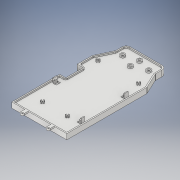
# Autodesk Inventor part: Display_Plate
Saved by Autodesk Inventor 2018 (Build 220112000, 112)
## iProperties
Created: 2019-05-28
Part Number: Display_Plate
Material: ABS Plastic
Document SubType Name: Modeling
Designer: Ash
Density: 1.06 g/cm^3
Appearance: Smooth - White
Author: Ash
Autodesk Inventor part; units mm, degrees
ref_plane "YZ Plane" through (0, 0, 0) normal (1, 0, 0) x (0, 1, 0)
ref_plane "XZ Plane" through (0, 0, 0) normal (0, 1, 0) x (-1, 0, 0)
ref_plane "XY Plane" through (0, 0, 0) normal (0, 0, 1) x (1, 0, 0)
sketch "Sketch1" plane through (0, 0, 0) normal (0, 1, 0) x (-1, 0, 0)
  line L0 (-80.01, -1.257939) -> (-80.01, -117.394059)
  line L1 (-80.01, -118.097939) -> (0, -118.097939) construction
  line L2 (0, -117.394059) -> (0, -96.380939)
  line L3 (-79.712527, -118.735872) -> (-69.512473, -140.609959)
  line L4 (-80.01, -118.097939) -> (-55.874615, -118.097939) construction
  line L5 (-0.297473, -118.735872) -> (-10.497527, -140.609959)
  line L6 (0, -118.097939) -> (24.135385, -118.097939) construction
  line L7 (-10.795, -141.247892) -> (-69.215, -141.247892) construction
  line L8 (-69.215, -141.951772) -> (-69.215, -150.645892)
  line L9 (-62.865, -156.995892) -> (-17.145, -156.995892)
  line L10 (-10.795, -150.645892) -> (-10.795, -141.951772)
  arc A0 (-0.297473, -118.735872) -> (0, -117.394059) centre (-3.175, -117.394059) ccw
  arc A1 (-80.01, -117.394059) -> (-79.712527, -118.735872) centre (-76.835, -117.394059) ccw
  arc A2 (-69.215, -150.645892) -> (-62.865, -156.995892) centre (-62.865, -150.645892) ccw
  arc A3 (-17.145, -156.995892) -> (-10.795, -150.645892) centre (-17.145, -150.645892) ccw
  arc A4 (-10.497527, -140.609959) -> (-10.795, -141.951772) centre (-7.62, -141.951772) ccw
  arc A5 (-69.215, -141.951772) -> (-69.512473, -140.609959) centre (-72.39, -141.951772) ccw
  line L11 (0, -96.380939) -> (-8.763, -96.380939)
  line L12 (-8.763, -96.380939) -> (-8.763, -70.980939)
  line L13 (-8.763, -70.980939) -> (0, -70.980939)
  line L14 (-80.01, -1.257939) -> (0, -1.257939)
  line L15 (0, -70.980939) -> (0, -1.257939)
  point P0 (0, 0)
  point P1 (-69.215, -156.995892)
  dimension "d0" = 80.01
  dimension "d1" = 116.84
  dimension "d3" = 65
  dimension "d4" = 115
  dimension "d5" = 58.42
  dimension "d6" = 15.748
  dimension "d7" = 3.175
  dimension "d8" = 6.35
  dimension "d9" = 3.175
  dimension "d45" = 8.763
  dimension "d46" = 25.4
  dimension "d47" = 21.717
  constraints: 32 end point, 12 point on circle, 12 point on line, 12 tangent, 6 centre point, 5 horizontal, 4 parallel, 4 perpendicular, 3 equal radius, 2 equal length, 1 horizontal alignment, 1 vertical
  measures "d0" distance of L1.end L1.start
  measures "d1" distance of L0.start L1.start
  measures "d3" angle of L3 L4
  measures "d4" angle of L5 L6
  measures "d5" distance of point (-69.215, -141.248) L7.start
  measures "d6" distance of point (-69.215, -156.996) L7.end
  measures "d7" radius of A0
  measures "d8" radius of A2
  measures "d9" radius of A4
  measures "d45" distance of L2.end L11.end
  measures "d46" distance of L11.end L12.end
  measures "d47" distance from line of L1.end L11
extrude "Extrusion1" add sketch "Sketch1" along normal blind 3.81
shell "Shell1" thickness 1.778 removed faces 1 at (56.261, 3.81, -63.210979)
sketch "Sketch2" plane through (1.778, 1.778, -1.778) normal (0, 1, 0) x (1, 0, 0)
  arc A0 (65.659, 140.173772) -> (66.123058, 138.080544) centre (70.612, 140.173772) ccw
  line L0 (65.776406, 139.101747) -> (60.579, 139.101747)
  line L1 (65.659, 148.867892) -> (65.659, 140.173772)
  line L2 (65.659, 140.625747) -> (60.579, 140.625747)
  line L3 (76.454, 115.616059) -> (76.454, 1.257939)
  arc A1 (76.454, 115.616059) -> (76.323112, 116.206456) centre (75.057, 115.616059) ccw
  line L4 (66.123058, 138.080544) -> (76.323112, 116.206456)
  arc A2 (65.659, 140.173772) -> (66.123058, 138.080544) centre (70.612, 140.173772) ccw
  line L5 (65.659, 148.867892) -> (65.659, 140.173772)
  arc A3 (65.659, 148.867892) -> (61.087, 153.439892) centre (61.087, 148.867892) ccw construction
  line L6 (15.367, 153.439892) -> (61.087, 153.439892) construction
  arc A4 (15.367, 153.439892) -> (10.795, 148.867892) centre (15.367, 148.867892) ccw construction
  line L7 (10.795, 140.173772) -> (10.795, 148.867892)
  arc A5 (10.330942, 138.080544) -> (10.795, 140.173772) centre (5.842, 140.173772) ccw
  line L8 (0.130888, 116.206456) -> (10.330942, 138.080544) construction
  arc A6 (0.130888, 116.206456) -> (0, 115.616059) centre (1.397, 115.616059) ccw
  line L9 (0, 96.380939) -> (0, 115.616059)
  circle A7 centre (57.235739, 139.863747) radius 1.905
  circle A8 centre (57.235739, 139.863747) radius 3.429
  line L10 (65.776406, 139.863747) -> (47.229764, 139.863747) construction
  line L11 (15.367, 153.439892) -> (61.087, 153.439892) construction
  line L12 (38.227, 153.439892) -> (38.227, -24.551353) construction
  line L13 (57.235739, 139.863747) -> (57.235739, 153.439892) construction
  line L14 (56.473739, 143.207008) -> (56.473739, 153.439892)
  line L15 (57.997739, 143.211092) -> (57.997739, 153.439892)
  line L16 (57.235739, 139.863747) -> (38.227, 145.482717) construction
  line L17 (57.235739, 139.863747) -> (38.227, 132.020717) construction
  circle A9 centre (38.227, 132.020717) radius 1.905
  circle A10 centre (38.227, 145.482717) radius 1.905
  circle A11 centre (38.227, 132.020717) radius 3.429
  circle A12 centre (38.227, 145.482717) radius 3.429
  line L18 (41.649128, 145.265732) -> (54.245625, 141.542217)
  line L19 (59.516104, 139.968345) -> (54.495452, 137.802468) construction
  line L20 (41.217114, 143.804247) -> (53.813611, 140.080731)
  line L21 (54.950087, 139.741356) -> (53.872726, 139.19428) construction
  line L22 (53.813611, 140.080731) -> (54.950087, 139.741356) construction
  line L23 (53.872726, 139.19428) -> (41.064475, 133.946016)
  line L24 (54.245625, 141.542217) -> (59.516104, 139.968345) construction
  line L25 (54.495452, 137.802468) -> (41.618556, 132.526076)
  line L26 (10.677594, 139.101747) -> (15.875, 139.101747)
  line L27 (10.795, 140.625747) -> (15.875, 140.625747)
  circle A13 centre (19.218261, 139.863747) radius 1.905
  circle A14 centre (19.218261, 139.863747) radius 3.429
  line L28 (19.980261, 143.207008) -> (19.980261, 153.439892)
  line L29 (18.456261, 143.211092) -> (18.456261, 153.439892)
  line L30 (34.804872, 145.265732) -> (22.208375, 141.542217)
  line L31 (35.236886, 143.804247) -> (22.640389, 140.080731)
  line L32 (22.581274, 139.19428) -> (35.389525, 133.946016)
  line L33 (21.958548, 137.802468) -> (34.835444, 132.526076)
  line L34 (34.835444, 132.526076) -> (21.958548, 137.802468)
  line L35 (22.581274, 139.19428) -> (35.389525, 133.946016)
  circle A15 centre (38.227, 132.020717) radius 3.429
  circle A16 centre (38.227, 145.482717) radius 3.429
  circle A17 centre (19.218261, 139.863747) radius 3.429
  line L36 (15.367, 153.439892) -> (61.087, 153.439892)
  line L37 (8.763, 96.380939) -> (0, 96.380939)
  line L38 (8.763, 67.424939) -> (8.763, 96.380939)
  line L39 (0, 67.424939) -> (8.763, 67.424939)
  line L40 (0, 1.257939) -> (0, 67.424939)
  line L41 (76.454, 1.257939) -> (0, 1.257939)
  point P0 (-1.778, -1.778)
  dimension "d13" = 1.524
  dimension "d14" = 5.08
  dimension "d15" = 3.81
  dimension "d16" = 1.524
  dimension "d17" = 0.762
  dimension "d20" = 1.524
  dimension "d21" = 0.762
  dimension "d22" = 13.462
  dimension "d23" = 3.81
  dimension "d24" = 3.81
  dimension "d25" = 1.524
  dimension "d26" = 1.524
  dimension "d27" = 0.762
  dimension "d28" = 0.762
  dimension "d30" = 1.524
  constraints: 54 end point, 17 symmetric about line, 7 centre point, 7 point on line, 6 point on circle, 5 coincident, 4 parallel, 2 horizontal, 2 vertical, 1 concentric, 1 midpoint, 1 perpendicular, 28 other
  measures "d13" distance between parallel lines of L0 L2
  measures "d14" distance of L2.start L2.end
  measures "d15" diameter of A7
  measures "d17" distance between parallel lines of L0 L10
  measures "d20" distance between parallel lines of L15 L14
  measures "d21" distance between parallel lines of L13 L14
  measures "d22" distance of L16.end L17.end
  measures "d23" diameter of A9
  measures "d24" diameter of A10
  measures "d25" radial gap between concentric circles of A9 A11
  measures "d26" radial gap between concentric circles of A10 A12
  measures "d27" distance between parallel lines of L16 L18
  measures "d28" distance between parallel lines of L16 L20
  measures "d30" distance between parallel lines of L25 L23
sketch "Sketch3" plane through (1.778, 1.778, -1.778) normal (0, 1, 0) x (1, 0, 0)
  circle A0 centre (19.218261, 139.748807) radius 1.905
  circle A1 centre (19.218261, 139.748807) radius 3.429
  circle A2 centre (38.227, 145.482717) radius 1.905
  circle A3 centre (38.227, 145.482717) radius 3.429
  circle A4 centre (38.227, 132.020717) radius 1.905
  circle A5 centre (38.227, 132.020717) radius 3.429
  circle A6 centre (57.235739, 139.748807) radius 1.905
  circle A7 centre (57.235739, 139.748807) radius 3.429
  arc A8 (60.579, 140.510807) -> (60.579, 140.510807) centre (57.235739, 139.748807) ccw
  line L0 (58.00154, 143.0912) -> (58.00154, 153.324952)
  line L1 (15.367, 153.439892) -> (61.087, 153.439892)
  line L2 (56.471752, 153.324952) -> (56.471752, 143.091615)
  line L3 (65.659, 148.867892) -> (65.659, 140.173772)
  arc A9 (65.659, 148.867892) -> (61.087, 153.439892) centre (61.087, 148.867892) ccw
  line L4 (15.367, 153.439892) -> (61.087, 153.439892)
  arc A10 (15.367, 153.439892) -> (10.795, 148.867892) centre (15.367, 148.867892) ccw
  line L5 (10.795, 140.173772) -> (10.795, 148.867892)
  arc A11 (10.330942, 138.080544) -> (10.795, 140.173772) centre (5.842, 140.173772) ccw
  line L6 (0.130888, 116.206456) -> (10.330942, 138.080544)
  arc A12 (0.130888, 116.206456) -> (0, 115.616059) centre (1.397, 115.616059) ccw
  line L7 (0, 96.380939) -> (0, 115.616059)
  line L8 (76.454, 115.616059) -> (76.454, 1.257939)
  arc A13 (76.454, 115.616059) -> (76.323112, 116.206456) centre (75.057, 115.616059) ccw
  line L9 (66.123058, 138.080544) -> (76.323112, 116.206456)
  arc A14 (65.659, 140.173772) -> (66.123058, 138.080544) centre (70.612, 140.173772) ccw
  line L10 (18.476733, 153.439892) -> (18.476733, 143.211608)
  circle A15 centre (19.218261, 139.748807) radius 3.429
  line L11 (19.95979, 143.096669) -> (19.95979, 153.439892)
  line L12 (22.199011, 141.443851) -> (34.80613, 145.246738)
  arc A16 (41.656, 145.482717) -> (41.656, 145.482717) centre (38.227, 145.482717) ccw
  line L13 (35.24625, 143.787673) -> (22.639132, 139.984786)
  line L14 (22.022965, 137.776073) -> (34.835444, 132.526076)
  arc A17 (41.656, 132.020717) -> (41.656, 132.020717) centre (38.227, 132.020717) ccw
  line L15 (22.600805, 139.186277) -> (35.389525, 133.946016)
  line L16 (15.875, 140.510807) -> (10.795, 140.510807)
  line L17 (10.795, 140.173772) -> (10.795, 148.867892)
  line L18 (15.875, 138.986807) -> (10.677594, 139.101747)
  line L19 (8.763, 96.380939) -> (0, 96.380939)
  line L20 (8.763, 67.424939) -> (8.763, 96.380939)
  line L21 (0, 67.424939) -> (8.763, 67.424939)
  line L22 (0, 1.257939) -> (0, 67.424939)
  line L23 (76.454, 1.257939) -> (0, 1.257939)
  point P0 (-1.778, -1.778)
  constraints: 20 end point, 7 point on circle, 3 point on line, 2 parallel, 2 vertical, 1 horizontal, 1 perpendicular, 9 other
sketch "Sketch5" plane through (1.778, 1.778, -1.778) normal (0, 1, 0) x (1, 0, 0)
  line L0 (0, 96.380939) -> (0, 115.616059)
  line L1 (0, 115.616059) -> (10.16, 115.616059) construction
  arc A0 (76.454, 115.616059) -> (76.323112, 116.206456) centre (75.057, 115.616059) ccw
  line L2 (76.323112, 116.206456) -> (66.163112, 116.206456) construction
  line L3 (-1.778, 69.202939) -> (-1.778, -1.778)
  line L4 (-1.778, 23.137892) -> (19.304, 23.137892) construction
  line L5 (-1.778, 23.137892) -> (19.304, 23.137892) construction
  line L6 (76.454, 23.137892) -> (55.372, 23.137892) construction
  line L7 (61.087, 155.217892) -> (15.367, 155.217892)
  line L8 (9.496281, 155.217892) -> (45.056281, 155.217892) construction
  line L9 (10.795, 140.510807) -> (22.647261, 140.510807) construction
  line L10 (10.16, 116.378059) -> (5.08, 116.378059)
  line L11 (5.08, 116.378059) -> (5.08, 114.854059)
  line L12 (5.08, 114.854059) -> (10.16, 114.854059)
  line L13 (10.16, 114.854059) -> (10.16, 116.378059)
  line L14 (6.858, 113.076059) -> (8.382, 113.076059)
  line L15 (8.382, 113.076059) -> (8.382, 118.156059)
  line L16 (8.382, 118.156059) -> (6.858, 118.156059)
  line L17 (6.858, 118.156059) -> (6.858, 113.076059)
  line L18 (6.858, 113.076059) -> (8.382, 118.156059) construction
  line L19 (8.382, 113.076059) -> (6.858, 118.156059) construction
  line L20 (7.62, 116.378059) -> (7.62, 114.854059) construction
  circle A1 centre (7.62, 115.616059) radius 0.889
  line L21 (68.703112, 115.444456) -> (63.623112, 115.444456)
  line L22 (63.623112, 115.444456) -> (63.623112, 116.968456)
  line L23 (63.623112, 116.968456) -> (68.703112, 116.968456)
  line L24 (68.703112, 116.968456) -> (68.703112, 115.444456)
  line L25 (65.401112, 113.666456) -> (66.925112, 113.666456)
  line L26 (66.925112, 113.666456) -> (66.925112, 118.746456)
  line L27 (66.925112, 118.746456) -> (65.401112, 118.746456)
  line L28 (65.401112, 118.746456) -> (65.401112, 113.666456)
  line L29 (65.401112, 113.666456) -> (66.925112, 118.746456) construction
  line L30 (66.925112, 113.666456) -> (65.401112, 118.746456) construction
  line L31 (66.163112, 115.444456) -> (66.163112, 116.968456) construction
  circle A2 centre (66.163112, 116.206456) radius 0.889
  line L32 (54.61, 20.597892) -> (56.134, 20.597892)
  line L33 (55.372, 22.375892) -> (55.372, 23.899892) construction
  line L34 (52.832, 23.899892) -> (57.912, 23.899892)
  circle A3 centre (55.372, 23.137892) radius 0.889
  line L35 (57.912, 23.899892) -> (57.912, 22.375892)
  line L36 (57.912, 22.375892) -> (52.832, 22.375892)
  line L37 (56.134, 20.597892) -> (56.134, 25.677892)
  line L38 (54.61, 20.597892) -> (56.134, 25.677892) construction
  line L39 (56.134, 20.597892) -> (54.61, 25.677892) construction
  line L40 (54.61, 25.677892) -> (54.61, 20.597892)
  line L41 (56.134, 25.677892) -> (54.61, 25.677892)
  line L42 (52.832, 22.375892) -> (52.832, 23.899892)
  line L43 (18.542, 20.597892) -> (20.066, 20.597892)
  line L44 (19.304, 22.375892) -> (19.304, 23.899892) construction
  line L45 (16.764, 23.899892) -> (21.844, 23.899892)
  circle A4 centre (19.304, 23.137892) radius 0.889
  line L46 (21.844, 23.899892) -> (21.844, 22.375892)
  line L47 (21.844, 22.375892) -> (16.764, 22.375892)
  line L48 (20.066, 20.597892) -> (20.066, 25.677892)
  line L49 (18.542, 20.597892) -> (20.066, 25.677892) construction
  line L50 (20.066, 20.597892) -> (18.542, 25.677892) construction
  line L51 (18.542, 25.677892) -> (18.542, 20.597892)
  line L52 (20.066, 25.677892) -> (18.542, 25.677892)
  line L53 (16.764, 22.375892) -> (16.764, 23.899892)
  line L54 (76.454, 115.616059) -> (76.454, 1.257939)
  line L55 (76.454, 0) -> (0, 0)
  point P0 (22.647261, 139.748807)
  point P1 (68.703112, 117.203559)
  point P2 (57.912, 118.791059)
  point P3 (55.372, 23.137892)
  point P4 (21.844, 120.378559)
  point P5 (19.304, 23.137892)
  point P6 (7.62, 115.616059)
  dimension "d48" = 10.16
  dimension "d49" = 10.16
  dimension "d50" = 21.082
  dimension "d52" = 21.082
  dimension "d56" = 0.762
  dimension "d57" = 0.762
  dimension "d58" = 5.08
  dimension "d59" = 1.524
  dimension "d60" = 5.08
  dimension "d61" = 1.778
  dimension "d66" = 5.08
  dimension "d67" = 1.524
  dimension "d68" = 5.08
  dimension "d69" = 1.778
  dimension "d70" = 1.524
  dimension "d71" = 5.08
  dimension "d72" = 1.524
  dimension "d73" = 5.08
  dimension "d74" = 1.778
  dimension "d75" = 1.524
  dimension "d76" = 5.08
  dimension "d77" = 1.524
  dimension "d78" = 5.08
  dimension "d79" = 1.778
  dimension "d80" = 1.524
  dimension "d160" = 132.08
  constraints: 100 end point, 27 midpoint, 16 parallel, 12 horizontal, 9 perpendicular, 9 point on line, 4 centre point, 4 coincident, 1 collinear
  measures "d48" distance of L0.end L1.end
  measures "d49" distance of L2.start L2.end
  measures "d50" distance of L4.end L4.start
  measures "d52" distance of L6.end L6.start
  measures "d56" distance between parallel lines of L1 L10
  measures "d57" distance between parallel lines of L1 L12
  measures "d58" distance between parallel lines of L13 L11
  measures "d59" distance of L16.end L15.end
  measures "d60" distance of L15.end L14.end
  measures "d61" diameter of A1
  measures "d66" distance between parallel lines of L24 L22
  measures "d67" distance of L30.end L26.end
  measures "d68" distance of L26.end L25.end
  measures "d69" diameter of A2
  measures "d70" distance between parallel lines of L21 L23
  measures "d71" distance between parallel lines of L35 L42
  measures "d72" distance of L41.end L37.end
  measures "d73" distance of L37.end L32.end
  measures "d74" diameter of A3
  measures "d75" distance between parallel lines of L36 L34
  measures "d76" distance between parallel lines of L46 L53
  measures "d77" distance of L52.end L48.end
  measures "d78" distance of L48.end L43.end
  measures "d79" diameter of A4
  measures "d80" distance between parallel lines of L47 L45
  measures "d160" distance between parallel lines of L7 L6
extrude "Extrusion7" add sketch "Sketch5" along normal blind 3.048 contours A1 L15 L12 L17 L10 | L10 A1 | A1 L15 | A1 L12 | L17 A1 | A2 L21 | L21 A2 L28 L23 L26 | L26 A2 | L23 A2 | A2 L28 | L36 A3 | A3 L40 L34 L37 L36 | A3 L40 | L37 A3 | A3 L34 | L47 A4 | A4 L51 L45 L48 L47 | A4 L51 | L48 A4 | A4 L45
extrude "Extrusion8" add sketch "Sketch5" along normal up to surface (2.032 mm away)
sketch "Sketch6" plane through (1.778, 1.778, -1.778) normal (0, 1, 0) x (1, 0, 0)
  line L0 (3.302, 61.074939) -> (7.366, 61.074939)
  line L1 (7.366, 61.074939) -> (7.366, 54.978939)
  line L2 (7.366, 54.978939) -> (3.302, 54.978939)
  line L3 (3.302, 54.978939) -> (3.302, 61.074939)
  line L4 (0, 67.424939) -> (8.763, 67.424939)
  line L5 (6.985, 69.202939) -> (-1.778, 69.202939)
  line L6 (-1.778, 69.202939) -> (-1.778, -1.778)
  line L7 (69.088, 29.718) -> (73.152, 29.718)
  line L8 (73.152, 29.718) -> (73.152, 23.622)
  line L9 (73.152, 23.622) -> (69.088, 23.622)
  line L10 (69.088, 23.622) -> (69.088, 29.718)
  line L11 (78.232, -0.520061) -> (78.232, 115.616059)
  line L12 (-1.778, -1.778) -> (78.232, -1.778)
  line L13 (69.088, 93.218) -> (73.152, 93.218)
  line L14 (73.152, 93.218) -> (73.152, 87.122)
  line L15 (73.152, 87.122) -> (69.088, 87.122)
  line L16 (69.088, 87.122) -> (69.088, 93.218)
  line L17 (76.454, 115.616059) -> (76.454, 1.257939)
  point P0 (0, 67.31)
  point P1 (76.454, 0)
  dimension "d82" = 4.064
  dimension "d83" = 6.096
  dimension "d85" = 8.128
  dimension "d86" = 5.08
  dimension "d87" = 4.064
  dimension "d88" = 6.096
  dimension "d89" = 5.08
  dimension "d90" = 25.4
  dimension "d91" = 4.064
  dimension "d92" = 6.096
  dimension "d93" = 88.9
  dimension "d95" = 5.08
  constraints: 24 end point, 6 parallel, 3 horizontal, 3 perpendicular, 1 other
  measures "d82" distance of L1.end L2.end
  measures "d83" distance of L0.end L1.end
  measures "d85" distance between parallel lines of L5 L0
  measures "d86" distance between parallel lines of L6 L3
  measures "d87" distance of L8.end L9.end
  measures "d88" distance of L7.end L8.end
  measures "d89" distance between parallel lines of L11 L8
  measures "d90" distance between parallel lines of L12 L9
  measures "d91" distance of L14.end L15.end
  measures "d92" distance of L13.end L14.end
  measures "d93" distance between parallel lines of L12 L15
  measures "d95" distance between parallel lines of L11 L14
extrude "Extrusion9" cut sketch "Sketch6" against normal through all
sketch "Sketch7" plane through (1.778, 1.778, -1.778) normal (0, 1, 0) x (1, 0, 0)
  line L0 (3.302, 54.978939) -> (3.302, 61.074939)
  line L1 (3.302, 60.439939) -> (2.032, 60.439939)
  line L2 (2.032, 60.439939) -> (2.032, 55.486939)
  line L3 (2.032, 55.486939) -> (3.302, 55.486939)
  line L4 (3.302, 55.486939) -> (3.302, 60.439939)
  line L5 (3.302, 61.074939) -> (7.366, 61.074939)
  line L6 (74.422, 92.583) -> (73.152, 92.583)
  line L7 (73.152, 92.583) -> (73.152, 87.63)
  line L8 (73.152, 87.63) -> (74.422, 87.63)
  line L9 (74.422, 87.63) -> (74.422, 92.583)
  line L10 (73.152, 93.218) -> (73.152, 87.122)
  line L11 (69.088, 93.218) -> (73.152, 93.218)
  line L12 (74.422, 29.21) -> (73.152, 29.21)
  line L13 (73.152, 29.21) -> (73.152, 24.257)
  line L14 (73.152, 24.257) -> (74.422, 24.257)
  line L15 (74.422, 24.257) -> (74.422, 29.21)
  line L16 (73.152, 29.718) -> (73.152, 23.622)
  line L17 (69.088, 29.718) -> (73.152, 29.718)
  line L18 (73.152, 23.622) -> (69.088, 23.622)
  point P0 (-1.778, -1.778)
  dimension "d98" = 1.27
  dimension "d99" = 4.953
  dimension "d100" = 0.635
  dimension "d103" = 1.27
  dimension "d104" = 4.953
  dimension "d105" = 0.635
  dimension "d106" = 1.27
  dimension "d107" = 4.953
  dimension "d109" = 0.635
  constraints: 24 end point, 6 parallel, 3 horizontal, 3 perpendicular, 2 collinear, 1 point on line
  measures "d98" distance of L3.end L2.end
  measures "d99" distance of L2.end L1.end
  measures "d100" distance between parallel lines of L5 L1
  measures "d103" distance of L8.end L7.end
  measures "d104" distance of L7.end L6.end
  measures "d105" distance between parallel lines of L11 L6
  measures "d106" distance of L14.end L13.end
  measures "d107" distance of L13.end L12.end
  measures "d109" distance between parallel lines of L18 L14
extrude "Extrusion10" add sketch "Sketch7" along normal blind 6.604
sketch "Sketch8" plane through (3.81, 1.778, -57.264939) normal (0, 0, 1) x (1, 0, 0)
  line L0 (1.27, 0) -> (1.27, 6.604) projected
  line L1 (1.27, 6.604) -> (2.286, 4.064)
  line L2 (2.286, 4.064) -> (1.27, 4.064)
  line L3 (0, 0) -> (0, 6.604) projected
  line L4 (0, 6.604) -> (1.27, 6.604) projected
  point P0 (-3.81, -1.778)
  dimension "d111" = 2.286
  dimension "d115" = 2.54
  constraints: 4 end point, 1 perpendicular, 1 point on line
  measures "d111" distance from line of L3 L1.end
  measures "d115" distance between parallel lines of L4 L2
extrude "Extrusion11" add sketch "Sketch8" against normal up to surface (4.953 mm away)
sketch "Sketch10" plane through (74.93, 1.778, -89.408) normal (0, 0, 1) x (1, 0, 0)
  line L0 (0, 0) -> (0, 6.604) projected
  line L1 (0, 6.604) -> (-1.016, 4.064)
  line L2 (-1.016, 4.064) -> (0, 4.064)
  line L3 (1.27, 0) -> (1.27, 6.604) projected
  line L4 (0, 6.604) -> (1.27, 6.604) projected
  point P0 (-74.93, -1.778)
  dimension "d114" = 2.286
  dimension "d116" = 2.54
  constraints: 4 end point, 1 horizontal, 1 point on line
  measures "d114" distance from line of L3 L1.end
  measures "d116" distance between parallel lines of L4 L2
sketch "Sketch11" plane through (74.93, 1.778, -26.035) normal (0, 0, 1) x (1, 0, 0)
  line L0 (0, 0) -> (0, 6.604) projected
  line L1 (0, 6.604) -> (-1.016, 4.064)
  line L2 (-1.016, 4.064) -> (0, 4.064)
  line L3 (1.27, 0) -> (1.27, 6.604) projected
  line L4 (0, 6.604) -> (1.27, 6.604) projected
  point P0 (-74.93, -1.778)
  dimension "d117" = 2.286
  dimension "d118" = 2.54
  constraints: 4 end point, 1 horizontal, 1 point on line
  measures "d117" distance from line of L3 L1.end
  measures "d118" distance between parallel lines of L4 L2
extrude "Extrusion12" add sketch "Sketch11" against normal up to surface (4.953 mm away)
extrude "Extrusion13" add sketch "Sketch10" against normal up to surface (4.953 mm away)
extrude "Extrusion14" cut sketch "Sketch3" against normal through all contours A0 | A2 | A4 | A6
sketch "Sketch12" plane through (0, 0, 0) normal (0, -1, 0) x (1, 0, 0)
  circle A0 centre (40.005, -133.798717) radius 1.905
  circle A1 centre (20.996261, -141.526807) radius 1.905
  circle A2 centre (40.005, -147.260717) radius 1.905
  circle A3 centre (59.013739, -141.526807) radius 1.905
  line L0 (70.866, -31.496) -> (70.866, -25.4)
  line L1 (70.866, -25.4) -> (74.93, -25.4)
  line L2 (74.93, -25.4) -> (74.93, -31.496)
  line L3 (74.93, -31.496) -> (70.866, -31.496)
  line L4 (5.08, -62.852939) -> (5.08, -56.756939)
  line L5 (5.08, -56.756939) -> (9.144, -56.756939)
  line L6 (9.144, -56.756939) -> (9.144, -62.852939)
  line L7 (9.144, -62.852939) -> (5.08, -62.852939)
  line L8 (70.866, -94.996) -> (70.866, -88.9)
  line L9 (70.866, -88.9) -> (74.93, -88.9)
  line L10 (74.93, -88.9) -> (74.93, -94.996)
  line L11 (74.93, -94.996) -> (70.866, -94.996)
  line L12 (0, -70.980939) -> (8.763, -70.980939)
  line L13 (8.763, -70.980939) -> (8.763, -96.380939)
  line L14 (8.763, -96.380939) -> (0, -96.380939)
  line L15 (0, -96.380939) -> (0, -117.394059)
  arc A4 (0, -117.394059) -> (0.297473, -118.735872) centre (3.175, -117.394059) ccw
  line L16 (0.297473, -118.735872) -> (10.497527, -140.609959)
  arc A5 (10.795, -141.951772) -> (10.497527, -140.609959) centre (7.62, -141.951772) ccw
  line L17 (10.795, -141.951772) -> (10.795, -150.645892)
  arc A6 (10.795, -150.645892) -> (17.145, -156.995892) centre (17.145, -150.645892) ccw
  line L18 (17.145, -156.995892) -> (62.865, -156.995892)
  arc A7 (62.865, -156.995892) -> (69.215, -150.645892) centre (62.865, -150.645892) ccw
  line L19 (69.215, -150.645892) -> (69.215, -141.951772)
  arc A8 (69.512473, -140.609959) -> (69.215, -141.951772) centre (72.39, -141.951772) ccw
  line L20 (69.512473, -140.609959) -> (79.712527, -118.735872)
  arc A9 (79.712527, -118.735872) -> (80.01, -117.394059) centre (76.835, -117.394059) ccw
  line L21 (80.01, -117.394059) -> (80.01, -1.257939)
  arc A10 (62.865, -155.725892) -> (67.945, -150.645892) centre (62.865, -150.645892) ccw
  line L22 (62.865, -155.725892) -> (17.145, -155.725892)
  arc A11 (12.065, -150.645892) -> (17.145, -155.725892) centre (17.145, -150.645892) ccw
  line L23 (12.065, -150.645892) -> (12.065, -141.951772)
  arc A12 (1.27, -117.394059) -> (1.448484, -118.199147) centre (3.175, -117.394059) ccw
  line L24 (1.27, -117.394059) -> (1.27, -97.650939)
  line L25 (1.27, -97.650939) -> (10.033, -97.650939)
  line L26 (10.033, -97.650939) -> (10.033, -69.710939)
  line L27 (10.033, -69.710939) -> (1.27, -69.710939)
  line L28 (1.27, -69.710939) -> (1.27, -1.384939)
  line L29 (1.27, -1.384939) -> (78.74, -1.384939)
  line L30 (78.74, -1.384939) -> (78.74, -117.394059)
  arc A13 (78.561516, -118.199147) -> (78.74, -117.394059) centre (76.835, -117.394059) ccw
  line L31 (78.561516, -118.199147) -> (69.215, -138.242816)
  line L32 (67.945, -141.951772) -> (67.945, -150.645892)
  line L33 (67.554406, -140.764807) -> (62.357, -140.764807)
  line L34 (67.945, -141.951772) -> (12.065, -141.951772) construction
  arc A14 (67.945, -133.257653) -> (62.865, -128.177653) centre (62.865, -133.257653) ccw
  line L35 (62.865, -128.177653) -> (17.145, -128.177653)
  arc A15 (17.145, -128.177653) -> (12.065, -133.257653) centre (17.145, -133.257653) ccw
  line L36 (12.065, -133.257653) -> (12.065, -141.951772)
  line L37 (67.945, -141.951772) -> (67.945, -133.257653)
  line L38 (10.795, -133.257653) -> (10.795, -141.951772)
  arc A16 (17.145, -126.907653) -> (10.795, -133.257653) centre (17.145, -133.257653) ccw
  line L39 (62.865, -126.907653) -> (17.145, -126.907653)
  arc A17 (69.215, -133.257653) -> (62.865, -126.907653) centre (62.865, -133.257653) ccw
  line L40 (69.215, -141.951772) -> (69.215, -133.257653)
  line L41 (10.795, -138.242816) -> (1.448484, -118.199147)
  line L42 (80.01, -1.257939) -> (0, -1.257939)
  line L43 (0, -1.257939) -> (0, -70.980939)
  point P0 (0, 0)
  point P1 (67.437, -142.288807)
  dimension "d125" = 1.27
  constraints: 38 end point, 16 point on circle, 12 symmetric about line, 8 centre point, 2 point on line, 12 other
  measures "d125" radial gap between concentric circles of A7 A10
extrude "Extrusion15" add sketch "Sketch12" along normal blind 4.064 contours L0 L1 L2 L3 | L4 L5 L6 L7 | L8 L9 L10 L11 | L43 L42 L21 A9 L20 A8 L40 L31 A13 L30 L29 L28 L27 L26 L25 L24 A12 L41 L38 A5 L16 A4 L15 L14 L13 L12 | L40 A17 L39 A16 L38 L41 A12 L24 L25 L26 L27 L28 L29 L30 A13 L31
sketch "Sketch13" plane through (0, 0, 0) normal (0, -1, 0) x (1, 0, 0)
  line L0 (76.2, -7.366) -> (9.144, -7.366)
  line L1 (9.144, -7.366) -> (9.144, -113.03)
  line L2 (9.144, -113.03) -> (76.2, -113.03)
  line L3 (76.2, -113.03) -> (76.2, -7.366)
  line L4 (0, 0) -> (80.01, 0)
  line L5 (80.01, -117.394059) -> (80.01, -1.257939)
  line L6 (77.724, -5.842) -> (7.62, -5.842)
  line L7 (7.62, -5.842) -> (7.62, -114.554)
  line L8 (7.62, -114.554) -> (77.724, -114.554)
  line L9 (77.724, -114.554) -> (77.724, -5.842)
  line L10 (77.724, -21.082) -> (76.2, -21.082)
  line L11 (70.104, -7.366) -> (70.104, -5.842)
  line L12 (9.144, -21.082) -> (7.62, -21.082)
  line L13 (15.24, -7.366) -> (15.24, -5.842)
  line L14 (77.724, -99.314) -> (76.2, -99.314)
  line L15 (70.104, -113.03) -> (70.104, -114.554)
  line L16 (15.24, -114.554) -> (15.24, -113.03)
  line L17 (9.144, -99.314) -> (7.62, -99.314)
  dimension "d128" = 67.056
  dimension "d129" = 105.664
  dimension "d130" = 7.366
  dimension "d131" = 3.81
  dimension "d132" = 1.524
  dimension "d133" = 15.24
  dimension "d134" = 7.62
  dimension "d135" = 7.62
  dimension "d136" = 15.24
  dimension "d137" = 15.24
  dimension "d138" = 7.62
  dimension "d139" = 15.24
  dimension "d140" = 7.62
  constraints: 32 end point, 16 point on line, 9 perpendicular, 5 parallel, 1 horizontal, 3 other
  measures "d128" distance of L2.end L1.end
  measures "d129" distance of L1.end L0.end
  measures "d130" distance between parallel lines of L4 L0
  measures "d131" distance between parallel lines of L5 L3
  measures "d132" distance between parallel lines of L3 L9
  measures "d133" distance between parallel lines of L6 L10
  measures "d134" distance between parallel lines of L9 L11
  measures "d135" distance between parallel lines of L7 L13
  measures "d136" distance between parallel lines of L6 L12
  measures "d137" distance between parallel lines of L8 L17
  measures "d138" distance between parallel lines of L7 L16
  measures "d139" distance between parallel lines of L8 L14
  measures "d140" distance between parallel lines of L9 L15
extrude "Extrusion16" add sketch "Sketch13" along normal blind 3.048 contours L0 L11 L6 L9 L10 L3 | L0 L1 L12 L7 L6 L13 | L14 L9 L8 L15 L2 L3 | L1 L2 L16 L8 L7 L17
fillet "Fillet1" radius 0.84582 4 edges at (56.261, 4.826, -24.9159) (20.193, 4.826, -24.9159) (8.509, 4.826, -117.3941) (67.0521, 4.826, -117.9845)
sketch "Sketch14" plane through (0, 3.81, 0) normal (0, 1, 0) x (1, 0, 0)
  circle A0 centre (21.209, -4.406261) radius 2.413
  line L0 (23.622, -4.406261) -> (23.622, 1.257939)
  line L1 (18.796, -4.406261) -> (18.796, 1.257939)
  circle A1 centre (21.209, -4.406261) radius 0.9525
  circle A2 centre (59.055, -4.406261) radius 2.413
  circle A3 centre (59.055, -4.406261) radius 0.9525
  line L2 (61.468, -4.406261) -> (61.468, 1.257939)
  line L3 (56.642, -4.406261) -> (56.642, 1.257939)
  line L4 (80.01, 1.257939) -> (80.01, 117.394059)
  line L5 (0, 1.257939) -> (80.01, 1.257939)
  line L6 (0, 70.980939) -> (0, 1.257939)
  dimension "d144" = 4.826
  dimension "d146" = 1.905
  dimension "d148" = 4.826
  dimension "d151" = 4.826
  dimension "d152" = 1.905
  dimension "d153" = 4.826
  dimension "d154" = 18.542
  dimension "d163" = 21.209
  dimension "d164" = 5.6642
  constraints: 8 end point, 4 centre point, 4 point on circle, 4 point on line, 3 parallel, 2 coincident, 2 vertical
  measures "d144" diameter of A0
  measures "d146" diameter of A1
  measures "d148" distance between parallel lines of L0 L1
  measures "d151" diameter of A2
  measures "d152" diameter of A3
  measures "d153" distance between parallel lines of L2 L3
  measures "d154" distance between parallel lines of L4 L2
  measures "d163" distance from line of L6 A0.centre
  measures "d164" distance from line of L5 A3.centre
extrude "Extrusion17" add sketch "Sketch14" against normal blind 2.286
fillet "Fillet2" radius 3.175 2 edges at (10.541, 2.794, -69.2029) (10.541, 2.794, -98.1589)
fillet "Fillet3" radius 3.175 1 edges at (1.778, 2.794, -98.1589)
extrude "Extrusion18" add sketch "Sketch2" along normal up to surface (2.032 mm away) contours A8 | A11 | A12 | A14
sketch "Sketch15" plane through (0, 0, 0) normal (0, -1, 0) x (1, 0, 0)
  line L0 (10.795, -133.257653) -> (10.795, -141.951772)
  line L1 (10.795, -141.951772) -> (10.795, -150.645892)
  arc A0 (10.795, -150.645892) -> (17.145, -156.995892) centre (17.145, -150.645892) ccw
  line L2 (17.145, -156.995892) -> (62.865, -156.995892)
  arc A1 (62.865, -156.995892) -> (69.215, -150.645892) centre (62.865, -150.645892) ccw
  line L3 (69.215, -150.645892) -> (69.215, -141.951772)
  line L4 (69.215, -141.951772) -> (69.215, -133.257653)
  arc A2 (69.215, -133.257653) -> (62.865, -126.907653) centre (62.865, -133.257653) ccw
  line L5 (62.865, -126.907653) -> (17.145, -126.907653)
  arc A3 (17.145, -126.907653) -> (10.795, -133.257653) centre (17.145, -133.257653) ccw
  circle A4 centre (40.005, -133.798717) radius 1.905
  circle A5 centre (20.996261, -141.526807) radius 1.905
  circle A6 centre (40.005, -147.260717) radius 1.905
  circle A7 centre (59.013739, -141.526807) radius 1.905
  line L6 (17.145, -128.431653) -> (62.865, -128.431653)
  arc A8 (67.691, -133.257653) -> (62.865, -128.431653) centre (62.865, -133.257653) ccw
  line L7 (67.691, -133.257653) -> (67.691, -141.951772)
  line L8 (67.691, -141.951772) -> (67.691, -150.645892)
  arc A9 (62.865, -155.471892) -> (67.691, -150.645892) centre (62.865, -150.645892) ccw
  line L9 (62.865, -155.471892) -> (17.145, -155.471892)
  arc A10 (12.319, -150.645892) -> (17.145, -155.471892) centre (17.145, -150.645892) ccw
  line L10 (12.319, -150.645892) -> (12.319, -141.951772)
  line L11 (12.319, -141.951772) -> (12.319, -133.257653)
  arc A11 (17.145, -128.431653) -> (12.319, -133.257653) centre (17.145, -133.257653) ccw
  point P0 (0, 0)
  dimension "d165" = 1.524
  constraints: 12 end point, 8 point on circle, 4 centre point, 9 other
  measures "d165" distance between parallel lines of L5 L6
extrude "Extrusion19" add sketch "Sketch15" along normal blind 4.572 contours A3 L5 A2 L4 L3 A1 L2 A0 L1 L0
body "Solid1"
